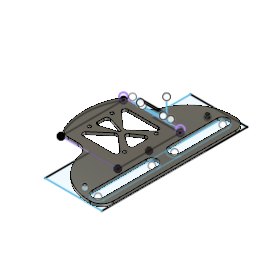
lidar_holder (Autodesk Fusion 360 design; units mm, degrees)
Autodesk Fusion 360 part; units mm, degrees
note: some values were not read from the file. Set by a fixed rule: which sketch regions a step uses.
sketch "Sketch1" plane through (0, 0, 0) normal (0, 0, 1) x (1, 0, 0)
  line L0 (0, 0) -> (100, 0)
  line L1 (100, 0) -> (100, 110)
  line L2 (100, 110) -> (0, 110)
  line L3 (0, 110) -> (0, 0)
  circle A0 centre (15, 35) radius 2.75
  circle A1 centre (15, 75) radius 2.75
  circle A2 centre (85, 83) radius 2.75
  circle A3 centre (85, 27) radius 2.75
  line L4 (85, 35) -> (85, 75)
  line L5 (15, 67.5) -> (15, 42.5)
  line L6 (85, 35) -> (55, 55)
  line L7 (85, 75) -> (55, 55)
  line L8 (50, 50) -> (10, 15)
  line L9 (10, 15) -> (90, 15)
  line L10 (90, 15) -> (50, 50)
  line L11 (50, 60) -> (90, 95)
  line L12 (90, 95) -> (10, 95)
  line L13 (10, 95) -> (50, 60)
  line L14 (15, 42.5) -> (54.5, 55)
  line L15 (54.5, 55) -> (15, 67.5)
  dimension "d1" = 5.5
  dimension "d2" = 5.5
  dimension "d3" = 5.5
  dimension "d4" = 5.5
  dimension "d5" = 40
  dimension "d6" = 56
  dimension "d7" = 70
  dimension "d9" = 100
  dimension "d10" = 110
  dimension "d11" = 27
  dimension "d12" = 15
  dimension "d63" = 15
  dimension "d66" = 15
  dimension "d67" = 7.5
  dimension "d68" = 7.5
  dimension "d72" = 15
  dimension "d73" = 15
  dimension "d76" = 50
  dimension "d77" = 10
  dimension "d78" = 10
  dimension "d80" = 56.31
  dimension "d81" = 56.31
  dimension "d140" = 10
  dimension "d141" = 41.186
  dimension "d142" = 41.186
  dimension "d143" = 72.44
  dimension "d152" = 35
  dimension "d153" = 35
  dimension "d154" = 35
  constraint horizontal L0
  constraint vertical L1
  constraint horizontal L2
  constraint vertical L3
  constraint coincident L0.start L3.end
  constraint vertical A0.centre A1.centre
  constraint vertical A2.centre A3.centre
  constraint vertical L4
  constraint vertical L5
  constraint horizontal L9
  constraint parallel L8 L11
  constraint parallel L10 L13
  constraint horizontal L6.end L14.end
  measures "d1" diameter of A0
  measures "d2" diameter of A1
  measures "d3" diameter of A2
  measures "d4" diameter of A3
  measures "d5" vertical distance of A0.centre A1.centre
  measures "d6" vertical distance of A2.centre A3.centre
  measures "d7" horizontal distance of A1.centre A2.centre
  measures "d9" distance of L1.end L2.end
  measures "d10" distance of L0.end L1.end
  measures "d11" distance of L2 A2.centre
  measures "d12" distance of L1 A3.centre
  measures "d63" distance of L1 L4
  measures "d66" distance of L3 L5
  measures "d67" distance of A0.centre L5.end
  measures "d68" distance of A1.centre L5.start
  measures "d72" distance of L0 L9
  measures "d73" distance of L2 L12
  measures "d76" distance of L2 L11.start
  measures "d77" distance of L3 L12.end
  measures "d78" distance of L3 L8.end
  measures "d80" angle of L4 L6
  measures "d81" angle of L4 L7
  measures "d140" distance of L1 L9.end
  measures "d141" angle of L12 L13
  measures "d142" angle of L11 L12
  measures "d143" angle of L5 L14
  measures "d152" distance of L2 L4.end
  measures "d153" distance of L0 L4.start
  measures "d154" distance of L2 A1.centre
extrude "Extrude13" add sketch "Sketch1" along normal blind 5
sketch "Sketch2" plane through (0, 110, 0) normal (0, 1, 0) x (-1, 0, 0)
  line L0 (-100, 0) -> (0, 0)
  line L1 (0, 0) -> (0, 10)
  line L2 (0, 10) -> (-100, 10)
  line L3 (-100, 10) -> (-100, 0)
  arc A0 (-29.9676, 8) -> (-29.9676, 14) centre (-29.9676, 11) ccw
  line L4 (-75.9121, 43) -> (-76, 43)
  line L5 (-29.9676, 8) -> (-33.1608, 8)
  line L6 (-29.9676, 14) -> (-69.9676, 14)
  line L7 (-69.9676, 8) -> (-29.9676, 8)
  arc A1 (-69.9676, 17) -> (-75.9676, 11) centre (-69.9676, 11) ccw
  line L8 (-69.9676, 17) -> (-29.9676, 17)
  line L9 (-76, 37.0055) -> (-75.9676, 11)
  arc A2 (-69.9676, 14) -> (-69.9676, 8) centre (-69.9676, 11) ccw
  arc A3 (-23.9676, 11) -> (-29.9676, 17) centre (-29.9676, 11) ccw
  line L10 (-23.9676, 5) -> (-75.9676, 5)
  line L11 (-75.9676, 5) -> (-83.3383, 5)
  line L12 (-23.9676, 5) -> (-17.9511, 5)
  arc A4 (-83.3383, 5) -> (-75.9676, 11) centre (-83.3383, 12.5273) ccw
  arc A5 (-23.9676, 11) -> (-17.9511, 5) centre (-16.0025, 12.9705) ccw
  line L13 (0, 5) -> (-100, 5)
  dimension "d108" = 6
  dimension "d109" = 6
  dimension "d110" = 3
  dimension "d111" = 40
  dimension "d112" = 6
  dimension "d115" = 6
  dimension "d116" = 40
  dimension "d119" = 6
  dimension "d120" = 52
  dimension "d121" = 3
  dimension "d135" = 12
  constraint tangent L6 A2
  constraint horizontal L6
  constraint horizontal L8
  constraint parallel L4 L8
  constraint concentric A1 A2
  constraint tangent A1 L9
  constraint coincident L8.start A1
  constraint coincident L9.start A1
  constraint coincident A1.start L8
  constraint concentric A0 A3
  constraint tangent L11 A4
  constraint horizontal L10
  measures "d108" diameter of A2
  measures "d109" diameter of A0
  measures "d110" distance of L6 L8
  measures "d111" distance of A0.end L6.end
  measures "d112" distance of A1.centre L9
  measures "d115" radius of A3
  measures "d116" distance of A1.centre A0.centre
  measures "d119" distance of A3.start L10.start
  measures "d120" distance of L10.start L10.end
  measures "d121" distance of L7 L10
  measures "d135" distance of L8 L13
extrude "Extrude14" add sketch "Sketch2" against normal blind 110 contours L2 A0 L5 L7 A2 L10 L11 L12 A4 A5 L13 | L2 A0 L6 A1 L8 A2 A3 A4 A5
sketch "Sketch6" plane through (0, 0, 22) normal (0, 0, 1) x (-1, 0, 0)
  line L0 (-70.0055, -110) -> (-30, -110)
  line L1 (-30, -110) -> (-30, 0)
  line L2 (-30, 0) -> (-70.0055, 0)
  line L3 (-70.0055, 0) -> (-70.0055, -110)
  line L4 (-10, -10) -> (-90, -10)
  line L5 (-90, -10) -> (-90, -100)
  line L6 (-90, -100) -> (-10, -100)
  line L7 (-10, -100) -> (-10, -10)
  line L8 (-69.9676, -110) -> (-29.9676, -110)
  line L9 (-100, 0) -> (-100, -110)
  line L10 (0, -110) -> (0, 0)
  dimension "d127" = 10
  dimension "d128" = 10
  dimension "d129" = 10
  dimension "d130" = 10
  constraint horizontal L4
  constraint vertical L5
  constraint horizontal L6
  constraint vertical L7
  measures "d127" distance of L6 L8
  measures "d128" distance of L2 L4
  measures "d129" distance of L5 L9
  measures "d130" distance of L7 L10
extrude "Extrude15" cut sketch "Sketch6" against normal blind 17 contours L3 L4 L5 L6 | L1 L3 L4 L6 | L1 L4 L6 L7
fillet "Fillet4" radius 2 1 edges at (54.5, 55, 2.5)
fillet "Fillet5" radius 5 3 edges at (50, 50, 2.5) (55, 55, 2.5) (50, 60, 2.5)
fillet "Fillet6" radius 5 6 edges at (10, 15, 2.5) (90, 15, 2.5) (85, 35, 2.5) (85, 75, 2.5) (90, 95, 2.5) (10, 95, 2.5)
fillet "Fillet7" radius 5 2 edges at (15, 67.5, 2.5) (15, 42.5, 2.5)
sketch "Sketch7" plane through (0, 0, 0) normal (0, 1, 0) x (1, 0, 0)
  line L0 (90, -5) -> (3.9374, -5)
  line L1 (3.9374, -5) -> (3.9374, -36.9823)
  line L2 (3.9374, -36.9823) -> (90, -36.9823)
  line L3 (90, -36.9823) -> (90, -5)
  constraint horizontal L0
  constraint vertical L1
  constraint horizontal L2
  constraint vertical L3
extrude "Extrude16" cut sketch "Sketch7" along normal blind 130
sketch "Sketch8" plane through (0, 0, 0) normal (0, 0, 1) x (1, 0, 0)
  circle A0 centre (100, 158) radius 2.5
  circle A1 centre (100, -58) radius 2.5
  line L0 (0, 0) -> (100, 0)
  line L1 (50, 110) -> (50, 178)
  line L2 (50, 178) -> (150, 178)
  line L3 (150, 178) -> (150, -78)
  line L4 (150, -78) -> (50, -78)
  line L5 (50, -78) -> (50, 0)
  line L6 (100, 0) -> (50, 0)
  line L7 (100, 0) -> (100, 110)
  line L8 (100, 110) -> (50, 110)
  line L9 (0, 0) -> (0, 110)
  arc A2 (0, 110) -> (0, 0) centre (100, 55) ccw
  arc A3 (97.7575, -59.1051) -> (102.2425, -59.1051) centre (100, 55) ccw
  line L10 (115, 160) -> (115, -60)
  line L11 (135, -60) -> (135, 160)
  arc A4 (135, 160) -> (115, 160) centre (125, 160) ccw
  arc A5 (115, -60) -> (135, -60) centre (125, -60) ccw
  arc A6 (135, 35) -> (115, 35) centre (125, 35) ccw
  arc A7 (115, 75) -> (135, 75) centre (125, 75) ccw
  point P0 (100, 110)
  dimension "d157" = 5
  dimension "d158" = 5
  dimension "d159" = 216
  dimension "d160" = 158
  dimension "d161" = 100
  dimension "d162" = 20
  dimension "d163" = 20
  dimension "d164" = 100
  dimension "d167" = 20
  dimension "d168" = 25
  constraint vertical L1
  constraint perpendicular L1 L2
  constraint perpendicular L2 L3
  constraint perpendicular L1 L4
  constraint midpoint L0 L5.end
  constraint perpendicular L0 L5
  constraint coincident L0.end L6.start
  constraint perpendicular L0 L7
  constraint perpendicular L1 L8
  constraint coincident P0 L7.end
  constraint midpoint L7 A2.centre
  constraint coincident L0.start A2
  constraint coincident L0.start L9.start
  constraint coincident L9.end A2.start
  constraint coincident A1 A3.start
  constraint concentric A2 A3
  constraint coincident L0 L9.start
  constraint coincident A1 A3.end
  constraint tangent L10 A5
  constraint parallel L3 L10
  constraint tangent L11 A4
  constraint perpendicular L2 L11
  constraint tangent L11 A6
  constraint tangent L11 A7
  constraint coincident L10 A6.end
  constraint coincident L11 A6.start
  constraint coincident L11 A7.end
  constraint coincident L10 A7.start
  measures "d157" diameter of A0
  measures "d158" diameter of A1
  measures "d159" distance of A0.centre A1.centre
  measures "d160" distance of A0.centre L0
  measures "d161" horizontal distance of A0.centre L9.end
  measures "d162" distance of A0.centre L2
  measures "d163" distance of A1.centre L4
  measures "d164" distance of L3.end L4.end
  measures "d167" diameter of A4
  measures "d168" distance of L3 A5.centre
extrude "Extrude20" add sketch "Sketch8" along normal blind 5 contours L0 L1 L2 L3 L4 L5 L6 L7 L8 | L9 A2 | L10 L11 A6 A7
fillet "Fillet10" radius 20 6 edges at (0, 0, 2.5) (50, 0, 2.5) (150, -78, 2.5) (0, 110, 2.5) (150, 178, 2.5) (50, 110, 2.5)
fillet "Fillet11" radius 80 2 edges at (50, 178, 2.5) (50, -78, 2.5)
equation "d160 = ( 216 / 2 ) * 1 mm + 50 mm"
